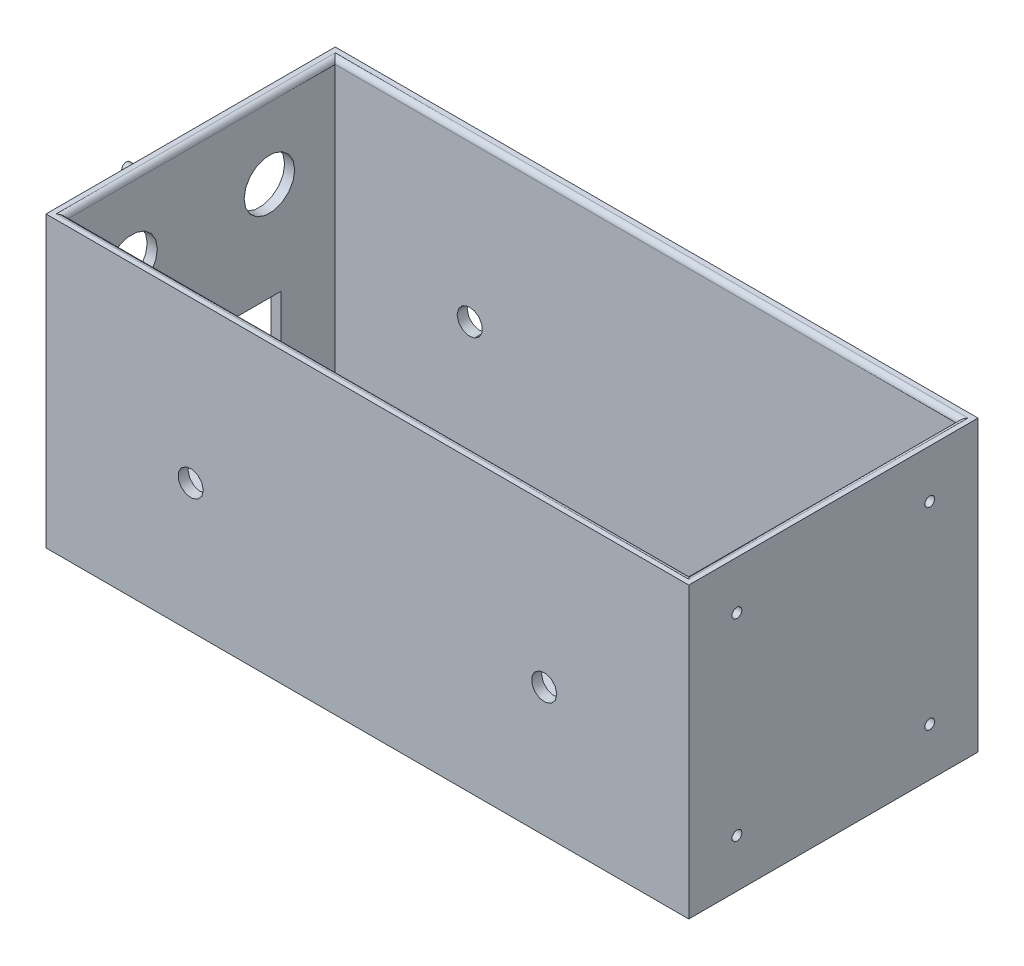
# Autodesk Inventor part: pranshu part
Saved by Autodesk Inventor 2022 (Build 260153070, 153G)
## iProperties
Created: 2021-06-28
Part Number: pranshu part
Material: PBT Plastic
Document SubType Name: Modeling
Designer: AKASH ARYAN
Density: 1.31 g/cm^3
Appearance: Smooth - White
Author: AKASH ARYAN
Autodesk Inventor part; units mm, degrees
ref_plane "YZ Plane" through (0, 0, 0) normal (1, 0, 0) x (0, 1, 0)
ref_plane "XZ Plane" through (0, 0, 0) normal (0, 1, 0) x (-1, 0, 0)
ref_plane "XY Plane" through (0, 0, 0) normal (0, 0, 1) x (1, 0, 0)
sketch "Sketch1" plane through (0, 0, 0) normal (1, 0, 0) x (0, 1, 0)
  point P0 (0, 0)
sketch "Sketch2" plane through (0, 0, 0) normal (1, 0, 0) x (0, 1, 0)
  line L0 (57.15, 57.15) -> (-57.15, 57.15)
  line L1 (-57.15, 57.15) -> (-57.15, -57.15)
  line L2 (-57.15, -57.15) -> (57.15, -57.15)
  line L3 (57.15, -57.15) -> (57.15, 57.15)
  line L4 (57.15, 57.15) -> (-57.15, -57.15) construction
  line L5 (-57.15, 57.15) -> (57.15, -57.15) construction
  point P0 (0, 0)
  dimension "d0" = 114.3
  dimension "d1" = 114.3
  constraints: 12 end point, 2 midpoint, 2 parallel, 1 horizontal, 1 perpendicular
  measures "d0" distance of L2.end L1.end
  measures "d1" distance of L1.end L0.end
extrude "Extrusion1" add sketch "Sketch2" along normal blind 254
sketch "Sketch3" plane through (0, 57.15, 57.15) normal (0, 1, 0) x (1, 0, 0)
  line L0 (3.9878, 110.3122) -> (250.0122, 110.3122)
  line L1 (250.0122, 110.3122) -> (250.0122, 3.9878)
  line L2 (250.0122, 3.9878) -> (3.9878, 3.9878)
  line L3 (3.9878, 3.9878) -> (3.9878, 110.3122)
  line L4 (0, 114.3) -> (254, 114.3) projected
  line L5 (0, 114.3) -> (0, 0) projected
  line L6 (0, 0) -> (254, 0) projected
  line L7 (254, 114.3) -> (254, 0) projected
  point P0 (0, 57.15)
  dimension "d4" = 3.9878
  dimension "d5" = 3.9878
  dimension "d6" = 3.9878
  dimension "d7" = 3.9878
  constraints: 8 end point, 2 parallel, 1 horizontal, 1 perpendicular
  measures "d4" distance between parallel lines of L4 L0
  measures "d5" distance between parallel lines of L5 L3
  measures "d6" distance between parallel lines of L6 L2
  measures "d7" distance between parallel lines of L7 L1
extrude "Extrusion2" cut sketch "Sketch3" against normal blind 110.3122 contours L0 L1 L2 L3
sketch "Sketch5" plane through (0, -57.15, 57.15) normal (0, 0, 1) x (1, 0, 0)
  circle A0 centre (57.15, 50.8) radius 5.0038
  circle A1 centre (196.85, 50.8) radius 5.0038
  line L0 (0, 0) -> (254, 0) projected
  line L1 (0, 114.3) -> (0, 0) projected
  line L2 (254, 114.3) -> (254, 0) projected
  point P0 (0, 57.15)
  dimension "d19" = 10.0076
  dimension "d20" = 10.0076
  dimension "d21" = 50.8
  dimension "d22" = 50.8
  dimension "d23" = 57.15
  dimension "d24" = 57.15
  constraints: 2 centre point
  measures "d19" diameter of A0
  measures "d20" diameter of A1
  measures "d21" distance from line of L0 A0.centre
  measures "d22" distance from line of L0 A1.centre
  measures "d23" distance from line of L1 A0.centre
  measures "d24" distance from line of L2 A1.centre
extrude "Extrusion3" cut sketch "Sketch5" against normal through all
sketch "Sketch6" plane through (0, -57.15, -57.15) normal (0, -1, 0) x (1, 0, 0)
  circle A0 centre (50.8, 57.15) radius 1.9939
  circle A1 centre (76.2, 57.15) radius 1.9939
  circle A2 centre (177.8, 57.15) radius 1.9939
  circle A3 centre (203.2, 57.15) radius 1.9939
  line L0 (0, 114.3) -> (254, 114.3) projected
  line L1 (0, 114.3) -> (0, 0) projected
  line L2 (254, 114.3) -> (254, 0) projected
  point P0 (0, 57.15)
  dimension "d27" = 3.9878
  dimension "d28" = 3.9878
  dimension "d29" = 3.9878
  dimension "d30" = 3.9878
  dimension "d31" = 57.15
  dimension "d32" = 57.15
  dimension "d33" = 57.15
  dimension "d34" = 57.15
  dimension "d35" = 50.8
  dimension "d36" = 50.8
  dimension "d37" = 76.2
  dimension "d38" = 76.2
  constraints: 4 centre point
  measures "d27" diameter of A0
  measures "d28" diameter of A1
  measures "d29" diameter of A2
  measures "d30" diameter of A3
  measures "d31" distance from line of L0 A0.centre
  measures "d32" distance from line of L0 A1.centre
  measures "d33" distance from line of L0 A2.centre
  measures "d34" distance from line of L0 A3.centre
  measures "d35" distance from line of L1 A0.centre
  measures "d36" distance from line of L2 A3.centre
  measures "d37" distance from line of L2 A2.centre
  measures "d38" distance from line of L1 A1.centre
extrude "Extrusion4" cut sketch "Sketch6" against normal through all
fillet "Fillet3" radius 1.999 4 edges at (250.0122, 57.15, 0) (127, 57.15, -53.1622) (127, 57.15, 53.1622) (3.9878, 57.15, 0)
sketch "Sketch7" plane through (0, 0, 0) normal (-1, 0, 0) x (0, 0, 1)
  circle A0 centre (-27.1526, 27.1526) radius 9.9949
  circle A1 centre (27.1526, 27.1526) radius 9.9949
  line L0 (-31.75, -11.7602) -> (31.75, -11.7602)
  line L1 (31.75, -11.7602) -> (31.75, -31.75)
  line L2 (31.75, -31.75) -> (-31.75, -31.75)
  line L3 (-31.75, -31.75) -> (-31.75, -11.7602)
  line L4 (57.15, -57.15) -> (-57.15, -57.15) projected
  line L5 (57.15, 57.15) -> (57.15, -57.15) projected
  line L6 (-57.15, 57.15) -> (57.15, 57.15) projected
  line L7 (-57.15, -57.15) -> (-57.15, 57.15) projected
  point P0 (0, 0)
  dimension "d43" = 19.9898
  dimension "d44" = 19.9898
  dimension "d45" = 63.5
  dimension "d46" = 19.9898
  dimension "d47" = 25.4
  dimension "d48" = 25.4
  dimension "d49" = 29.9974
  dimension "d50" = 29.9974
  dimension "d51" = 29.9974
  dimension "d52" = 29.9974
  constraints: 8 end point, 2 centre point, 2 parallel, 1 horizontal, 1 perpendicular
  measures "d43" diameter of A0
  measures "d44" diameter of A1
  measures "d45" distance of L1.end L2.end
  measures "d46" distance of L0.end L1.end
  measures "d47" distance between parallel lines of L2 L4
  measures "d48" distance between parallel lines of L5 L1
  measures "d49" distance from line of L5 A1.centre
  measures "d50" distance from line of A1.centre L6
  measures "d51" distance from line of L6 A0.centre
  measures "d52" distance from line of A0.centre L7
sketch "Sketch8" plane through (0, 0, 0) normal (-1, 0, 0) x (0, 0, 1)
  point P0 (0, 0)
extrude "Extrusion5" cut sketch "Sketch7" against normal blind 3.9878 contours A0 | A1 | L0 L1 L2 L3
sketch "Sketch9" plane through (254, 0, 0) normal (1, 0, 0) x (0, 0, -1)
  circle A0 centre (-38.1, 38.1) radius 1.9939
  circle A1 centre (38.1, 38.1) radius 1.9939
  circle A2 centre (-38.1, -38.1) radius 1.9939
  circle A3 centre (38.1, -38.1) radius 1.9939
  line L0 (57.15, 57.15) -> (-57.15, 57.15) projected
  line L1 (-57.15, 57.15) -> (-57.15, -57.15) projected
  line L2 (57.15, -57.15) -> (57.15, 57.15) projected
  line L3 (-57.15, -57.15) -> (57.15, -57.15) projected
  point P0 (0, 0)
  dimension "d55" = 3.9878
  dimension "d56" = 3.9878
  dimension "d57" = 3.9878
  dimension "d58" = 3.9878
  dimension "d59" = 19.05
  dimension "d60" = 19.05
  dimension "d61" = 19.05
  dimension "d62" = 19.05
  dimension "d63" = 19.05
  dimension "d64" = 19.05
  dimension "d65" = 19.05
  dimension "d66" = 19.05
  constraints: 4 centre point
  measures "d55" diameter of A0
  measures "d56" diameter of A1
  measures "d57" diameter of A2
  measures "d58" diameter of A3
  measures "d59" distance from line of L0 A0.centre
  measures "d60" distance from line of L1 A0.centre
  measures "d61" distance from line of L0 A1.centre
  measures "d62" distance from line of L2 A1.centre
  measures "d63" distance from line of L1 A2.centre
  measures "d64" distance from line of L3 A2.centre
  measures "d65" distance from line of L2 A3.centre
  measures "d66" distance from line of L3 A3.centre
sketch "Sketch10" plane through (254, 0, 0) normal (1, 0, 0) x (0, 0, -1)
  point P0 (0, 0)
extrude "Extrusion6" cut sketch "Sketch9" against normal blind 3.9878 contours A0 | A1 | A2 | A3
sketch "Sketch16" plane through (0, -57.15, 57.15) normal (0, 0, 1) x (1, 0, 0)
  point P0 (0, 57.15)
sketch "Sketch17" plane through (0, -57.15, 57.15) normal (0, 0, 1) x (1, 0, 0)
  point P0 (0, 57.15)
sketch "Sketch18" plane through (0, 0, 0) normal (-1, 0, 0) x (0, 0, 1)
  circle A0 centre (0, 31.75) radius 1.9939
  circle A1 centre (0, -44.45) radius 1.9939
  line L0 (-57.15, 57.15) -> (57.15, 57.15) projected
  line L1 (57.15, -57.15) -> (-57.15, -57.15) projected
  point P0 (0, 0)
  dimension "d89" = 3.9878
  dimension "d90" = 3.9878
  dimension "d91" = 25.4
  dimension "d92" = 12.7
  constraints: 2 centre point
  measures "d89" diameter of A0
  measures "d90" diameter of A1
  measures "d91" distance from line of L0 A0.centre
  measures "d92" distance from line of L1 A1.centre
extrude "Extrusion11" add sketch "Sketch18" along normal blind 25.4
sketch "Sketch19" plane through (0, 0, 0) normal (-1, 0, 0) x (0, 0, 1)
  point P0 (0, 0)
body "Solid1"
